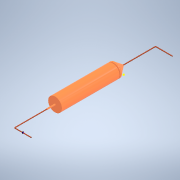
# Autodesk Inventor part: K50 – 29
Saved by Autodesk Inventor 2020.2 (Build 242310000, 310)
## iProperties
Created: 2020-03-29
Part Number: K50 – 29
Material: Copper
Document SubType Name: Modeling
Designer: IAmIllusion
Density: 8.94 g/cm^3
Appearance: Copper - Satin
Author: IAmIllusion
Autodesk Inventor part; units mm, degrees
ref_plane "YZ Plane" through (0, 0, 0) normal (1, 0, 0) x (0, 1, 0)
ref_plane "XZ Plane" through (0, 0, 0) normal (0, 1, 0) x (-1, 0, 0)
ref_plane "XY Plane" through (0, 0, 0) normal (0, 0, 1) x (1, 0, 0)
sketch "Sketch1" plane through (0, 0, 0) normal (0, 1, 0) x (-1, 0, 0)
  line L0 (4.5, 42) -> (4, 42)
  line L1 (-5.9955, 62) -> (-5.9955, 61.75)
  line L2 (-5.9955, 62) -> (-5.9955, 62.25)
  line L3 (4.25, 42) -> (4.25, 61.7)
  arc A0 (4.25, 61.7) -> (3.95, 62) centre (3.95, 61.7) ccw
  line L4 (3.95, 62) -> (-1.05, 62)
  point P0 (0, 0)
  constraints: 10 end point, 3 vertical, 2 horizontal, 2 point on circle, 1 centre point, 1 midpoint, 1 tangent
sketch "Sketch3" plane through (0, 0, 0) normal (1, 0, 0) x (0, 1, 0)
  circle A0 centre (0, -25.0051) radius 0.25
  point P0 (0, 0)
  constraints: 1 centre point
sketch "Sketch5" plane through (0, 0, 0) normal (0, 1, 0) x (-1, 0, 0)
  line L0 (8.5, 37) -> (0, 37)
  line L1 (4.0039, 37) -> (3.3039, 37)
  line L2 (0, 37) -> (4.25, 37)
  line L3 (4.25, 42) -> (3.85, 42)
  line L4 (4.25, 42) -> (4.65, 42)
  line L5 (4.65, 42) -> (4.65, 37)
  line L6 (3.85, 42) -> (3.85, 37)
  line L7 (4.25, 42) -> (4, 42)
  line L8 (4.25, 42) -> (4.5, 42)
  line L9 (4.5, 42) -> (4.5, 61.7)
  line L10 (4.2, 62) -> (4.0045, 62)
  line L11 (4.5024, -5) -> (3.9976, -5)
  line L12 (4.7401, -4.883) -> (8.5, 0)
  line L13 (3.7599, -4.883) -> (0, 0)
  line L14 (4.25, -5) -> (4, -5)
  line L15 (4.25, -5) -> (4.5066, -5)
  line L16 (4.25, -5) -> (4.5066, -5)
  line L17 (4.5066, -5) -> (4.5066, -24.7)
  line L18 (4.2066, -25) -> (4.0066, -25)
  line L19 (4.25, 0.9) -> (7.75, 0.9)
  line L20 (4.25, 0.9) -> (0.75, 0.9)
  line L21 (7.75, 0.9) -> (7.75, 1.3)
  line L22 (7.75, 1.3) -> (0.75, 1.3)
  line L23 (0.75, 1.3) -> (0.75, 0.9)
  line L24 (0.75, 0.9) -> (0, 0.9)
  line L25 (7.75, 0.9) -> (8.5, 0.9)
  line L26 (7.75, 1.3) -> (8.5, 1.3)
  line L27 (0.75, 1.3) -> (0, 1.3)
  line L28 (8.5, 37) -> (8.5, 1.3)
  line L29 (0, 37) -> (0, 1.3)
  line L30 (8.5, 0.9) -> (8.5, 0)
  line L31 (0, 0.9) -> (0, 0)
  arc A0 (4.5024, -5) -> (4.7401, -4.883) centre (4.5024, -4.7) ccw
  arc A1 (3.7599, -4.883) -> (3.9976, -5) centre (3.9976, -4.7) ccw
  line L32 (3.6976, -24.5) -> (-5.9934, -24.5)
  line L33 (4.0066, -25) -> (-5.9934, -25)
  line L34 (-5.9934, -25) -> (-5.9934, -24.5)
  line L35 (3.9976, -24.2) -> (3.9976, -5)
  line L36 (3.7, 61.5) -> (-5.9955, 61.5)
  line L37 (-5.9955, 61.5) -> (-5.9955, 62)
  line L38 (-5.9955, 62) -> (4.0045, 62)
  line L39 (4, 61.2) -> (4, 42)
  line L40 (4.25, 37) -> (4.25, 1.3)
  line L41 (4.25, 1.3) -> (4.25, -5)
  line L42 (4.25, 37) -> (4.25, 42)
  line L43 (4.25, 42) -> (4.25, 61.5)
  arc A2 (4.25, 61.5) -> (3.9684, 61.75) centre (3.892, 61.3803) ccw
  line L44 (3.9684, 61.75) -> (-5.9955, 61.75)
  arc A3 (4.5, 61.7) -> (4.2, 62) centre (4.2, 61.7) ccw
  arc A4 (4, 61.2) -> (3.7, 61.5) centre (3.7, 61.2) ccw
  line L45 (4.25, -5) -> (4.25, -24.5071)
  arc A5 (3.9999, -24.75) -> (4.25, -24.5071) centre (4.007, -24.5071) ccw
  line L46 (3.9999, -24.75) -> (-5.9934, -24.75)
  arc A6 (3.6976, -24.5) -> (3.9976, -24.2) centre (3.6976, -24.2) ccw
  arc A7 (4.2066, -25) -> (4.5066, -24.7) centre (4.2066, -24.7) ccw
  constraints: 94 end point, 16 point on circle, 13 tangent, 8 centre point, 8 vertical, 7 perpendicular, 7 point on line, 5 horizontal, 5 midpoint, 5 parallel, 2 collinear, 1 equal radius
sketch "Sketch6" plane through (0, 0, 0) normal (0, 1, 0) x (-1, 0, 0)
  line L0 (4.2294, -4.9987) -> (4.2294, -24.7)
  line L1 (3.9247, -25.0047) -> (-1.1526, -25.0047)
  arc A0 (3.9247, -25.0047) -> (4.2294, -24.7) centre (3.9247, -24.7) ccw
  constraints: 4 end point, 2 point on circle, 2 tangent, 1 centre point
sketch "Sketch7" plane through (0, 0, 0) normal (1, 0, 0) x (0, 1, 0)
  circle A0 centre (0, 62.0031) radius 0.2458
  point P0 (0, 0)
  point P1 (0, 0)
  constraints: 1 centre point
revolve "Revolution1" add sketch "Sketch5" angle 360 about axis through (-4.25, 0, 37) along (0, 0, -1) contours L28 L26 L22 L40 L0 | L0 L42 L4 L5 | L21 L19 L41 L22 | L25 L30 L12 A0 L15 L11 L41 L19
sweep "Sweep4" add profiles "Sketch7" path "Sketch1" separate body path curves L4 A0 L3
fillet "Fillet1" radius 0.2 2 edges at (0, 0, 0.9) (0, 0, 1.3)
sketch "Sketch8" plane through (1.05, 0, 62.0031) normal (1, 0, 0) x (0, 0, -1)
  circle A0 centre (0, 0) radius 0.2458 projected
  circle A1 centre (0, 0) radius 0.2458
  point P0 (62.0031, 0)
  constraints: 1 centre point, 1 coincident
extrude "Extrusion1" add sketch "Sketch8" along normal blind 5 bodies 2
sweep "Sweep5" add profiles "Sketch3" path "Sketch6" separate body
sketch "Sketch10" plane through (1.1526, 0, -25.0051) normal (1, 0, 0) x (0, 0, -1)
  circle A0 centre (0, 0) radius 0.25
  point P0 (-25.0051, 0)
  constraints: 1 centre point
extrude "Extrusion3" add sketch "Sketch10" along normal blind 5 bodies 3
body "Solid1"
body "Solid5"
body "Solid6"
